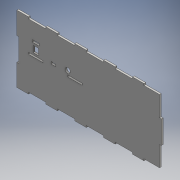
# Autodesk Inventor part: latPort
Saved by Autodesk Inventor 2016 (Build 200138000, 138)
## iProperties
Created: 2016-12-12
Part Number: latPort
Material: Generic
Document SubType Name: Modeling
Designer: NacostaMobile
Density: 1 g/cm^3
Appearance: Default
Author: NacostaMobile
Autodesk Inventor part; units mm, degrees
ref_plane "YZ Plane" through (0, 0, 0) normal (1, 0, 0) x (0, 1, 0)
ref_plane "XZ Plane" through (0, 0, 0) normal (0, 1, 0) x (-1, 0, 0)
ref_plane "XY Plane" through (0, 0, 0) normal (0, 0, 1) x (1, 0, 0)
sketch "Sketch1" plane through (0, 0, 0) normal (0, 1, 0) x (-1, 0, 0)
  line L0 (0, 0) -> (0, -3)
  line L1 (-250, -38) -> (-250, -78)
  line L2 (0, 0) -> (-20, 0)
  line L3 (-50, 0) -> (-50, -3)
  line L4 (-50, 0) -> (-70, 0)
  line L5 (-70, 0) -> (-70, -3)
  line L6 (-100, 0) -> (-100, -3)
  line L7 (-100, 0) -> (-120, 0)
  line L8 (-120, 0) -> (-120, -3)
  line L9 (-150, 0) -> (-150, -3)
  line L10 (-150, 0) -> (-170, 0)
  line L11 (-170, 0) -> (-170, -3)
  line L12 (-200, 0) -> (-200, -3)
  line L13 (-200, 0) -> (-220, 0)
  line L14 (-220, 0) -> (-220, -3)
  line L15 (-20, 0) -> (-20, -3)
  line L16 (-250, -58) -> (-250, -78)
  line L17 (-250, -78) -> (-247, -78)
  line L18 (-247, -78) -> (-247, -113)
  line L19 (-250, -58) -> (-250, -38)
  line L20 (-250, -38) -> (-247, -38)
  line L21 (-247, -38) -> (-247, -3)
  line L22 (-220, -3) -> (-247, -3)
  line L23 (-170, -3) -> (-200, -3)
  line L24 (-120, -3) -> (-150, -3)
  line L25 (-20, -3) -> (-50, -3)
  line L26 (-70, -3) -> (-100, -3)
  line L27 (0, -116) -> (0, -113)
  line L28 (0, -116) -> (-20, -116)
  line L29 (-50, -116) -> (-50, -113)
  line L30 (-50, -116) -> (-70, -116)
  line L31 (-70, -116) -> (-70, -113)
  line L32 (-100, -116) -> (-100, -113)
  line L33 (-100, -116) -> (-120, -116)
  line L34 (-120, -116) -> (-120, -113)
  line L35 (-150, -116) -> (-150, -113)
  line L36 (-150, -116) -> (-170, -116)
  line L37 (-170, -116) -> (-170, -113)
  line L38 (-200, -116) -> (-200, -113)
  line L39 (-200, -116) -> (-220, -116)
  line L40 (-220, -116) -> (-220, -113)
  line L41 (-20, -116) -> (-20, -113)
  line L42 (-3, -58) -> (-3, -78)
  line L43 (-3, -78) -> (0, -78)
  line L44 (-3, -58) -> (-3, -38)
  line L45 (-3, -38) -> (0, -38)
  line L46 (0, -113) -> (0, -78)
  line L47 (0, -38) -> (0, -3)
  line L48 (-50, -113) -> (-20, -113)
  line L49 (-100, -113) -> (-70, -113)
  line L50 (-150, -113) -> (-120, -113)
  line L51 (-247, -113) -> (-220, -113)
  line L52 (-200, -113) -> (-170, -113)
  line L53 (-20, -53) -> (-20, -56)
  line L54 (-20, -56) -> (-45, -56)
  line L55 (-45, -56) -> (-45, -53)
  line L56 (-113, -53) -> (-113, -56)
  line L57 (-113, -56) -> (-88, -56)
  line L58 (-88, -56) -> (-88, -53)
  line L59 (-20, -53) -> (-45, -53)
  line L60 (-88, -53) -> (-113, -53)
  line L61 (-63, -51) -> (-66.9, -51)
  line L62 (-66.9, -51) -> (-66.9, -47.1)
  line L63 (-66.9, -47.1) -> (-59.1, -47.1)
  line L64 (-59.1, -47.1) -> (-59.1, -51)
  line L65 (-59.1, -51) -> (-63, -51)
  circle A0 centre (-88, -46.5) radius 4.5
  line L66 (-37, -49.5) -> (-28, -49.5)
  line L67 (-28, -49.5) -> (-28, -38.5)
  line L68 (-28, -38.5) -> (-37, -38.5)
  line L69 (-37, -38.5) -> (-37, -49.5)
  line L70 (-32.5, -38.5) -> (-32.5, -38)
  line L71 (-32.5, -34.5) -> (-26.7, -34.5)
  line L72 (-26.7, -34.5) -> (-26.7, -30.5)
  line L73 (-26.7, -30.5) -> (-38.3, -30.5)
  line L74 (-38.3, -30.5) -> (-38.3, -34.5)
  line L75 (-38.3, -34.5) -> (-32.5, -34.5)
  dimension "d2" = 110
  dimension "d3" = 20
  dimension "d4" = 20
  dimension "d5" = 20
  dimension "d7" = 20
  dimension "d8" = 20
  dimension "d9" = 20
  dimension "d10" = 3
  dimension "d11" = 20
  dimension "d12" = 3
  dimension "d13" = 250
  dimension "d14" = 30
  dimension "d15" = 30
  dimension "d16" = 30
  dimension "d17" = 30
  dimension "d25" = 25
  dimension "d26" = 25
  dimension "d27" = 17
  dimension "d29" = 110
  dimension "d30" = 43
  dimension "d31" = 57
  dimension "d32" = 3
  dimension "d37" = 3.9
  dimension "d38" = 7.8
  dimension "d39" = 60
  dimension "d40" = 2
  dimension "d44" = 9
  dimension "d46" = 78
  dimension "d47" = 3
  dimension "d48" = 6.5
  dimension "d49" = 3
  dimension "d50" = 3
  dimension "d51" = 11
  dimension "d52" = 53
  dimension "d53" = 2
  dimension "d55" = 3.5
  dimension "d57" = 8
  dimension "d58" = 25
  dimension "d60" = 4
  dimension "d62" = 4
  dimension "d63" = 11.6
  dimension "d64" = 9
  constraints: 152 end point, 89 perpendicular, 10 point on line, 9 parallel, 4 horizontal, 4 vertical, 2 midpoint, 1 centre point
  measures "d2" distance of L21.end L18.end
  measures "d3" distance of L0.start L2.end
  measures "d4" distance of L3.start L4.end
  measures "d5" distance of L6.start L7.end
  measures "d7" distance of L9.start L10.end
  measures "d8" distance of L12.start L13.end
  measures "d9" distance of L1.end L16.start
  measures "d10" distance of L1.end L17.end
  measures "d11" distance of L1.start L16.start
  measures "d12" distance of L1.start L20.end
  measures "d13" distance between parallel lines of L46 L1
  measures "d14" distance of L15.end L3.end
  measures "d15" distance of L5.end L6.end
  measures "d16" distance of L8.end L9.end
  measures "d17" distance of L11.end L12.end
  measures "d25" distance of L53.end L54.end
  measures "d26" distance of L56.end L57.end
  measures "d27" distance between parallel lines of L44 L53
  measures "d29" distance between parallel lines of L44 L56
  measures "d30" distance between parallel lines of L58 L55
  measures "d31" distance between parallel lines of L49 L57
  measures "d32" distance between parallel lines of L42 L46
  measures "d37" distance of L61.end L62.end
  measures "d38" distance of L62.end L63.end
  measures "d39" distance from line of L44 L61.start
  measures "d40" distance between parallel lines of L60 L61
  measures "d44" diameter of A0
  measures "d46" distance between parallel lines of L28 L45
  measures "d47" distance of L54.end L55.end
  measures "d48" distance of A0.centre L58.end
  measures "d49" distance of L44.end L45.end
  measures "d50" distance of L13.end L14.end
  measures "d51" distance of L67.end L66.end
  measures "d52" distance between parallel lines of L57 L26
  measures "d53" distance from line of L54 L42.start
  measures "d55" distance between parallel lines of L59 L66
  measures "d57" distance between parallel lines of L69 L55
  measures "d58" distance from line of L56 A0.centre
  measures "d60" distance of L70.start L71.start
  measures "d62" distance of L71.end L72.end
  measures "d63" distance of L72.end L73.end
  measures "d64" distance of L66.start L66.end
extrude "Extrusion3" add sketch "Sketch1" along normal blind 3
body "Solid3"
